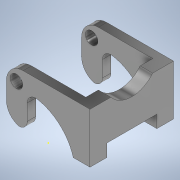
# Autodesk Inventor part: Peça 9
Saved by Autodesk Inventor 2021 (Build 250183000, 183)
## iProperties
Created: 2020-11-15
Part Number: Peça 9
Material: Liga de Nickel-Copper 400
Document SubType Name: Modeling
Designer: Bruno
Density: 8.83 g/cm^3
Appearance: Cromado - Preto polido
Author: Bruno
Autodesk Inventor part; units mm, degrees
ref_plane "YZ Plane" through (0, 0, 0) normal (1, 0, 0) x (0, 1, 0)
ref_plane "XZ Plane" through (0, 0, 0) normal (0, 1, 0) x (-1, 0, 0)
ref_plane "XY Plane" through (0, 0, 0) normal (0, 0, 1) x (1, 0, 0)
sketch "Esboço1" plane through (0, 0, 0) normal (0, 1, 0) x (-1, 0, 0)
  line L0 (-5, 5) -> (5, 5)
  line L1 (5, 5) -> (5, -5)
  line L2 (5, -5) -> (-5, -5)
  line L3 (-5, -5) -> (-5, 5)
  line L4 (-5, 5) -> (5, -5) construction
  line L5 (5, 5) -> (-5, -5) construction
  point P0 (0, 0)
  dimension "d0" = 10
  dimension "d1" = 10
  constraints: 12 end point, 2 midpoint, 2 parallel, 1 horizontal, 1 perpendicular
  measures "d0" distance between parallel lines of L2 L0
  measures "d1" distance between parallel lines of L3 L1
extrude "Extrusão1" add sketch "Esboço1" along normal blind 6
sketch "Esboço2" plane through (5, 0, 5) normal (1, 0, 0) x (0, 0, -1)
  line L0 (2, 0) -> (2, 1.5)
  line L1 (0, 0) -> (0, 6) projected
  line L2 (2, 1.5) -> (8, 1.5)
  line L3 (8, 1.5) -> (8, 0)
  line L4 (10, 0) -> (10, 6) projected
  line L5 (0, 0) -> (10, 0) projected
  point P0 (5, 0)
  dimension "d4" = 2
  dimension "d5" = 1.5
  dimension "d6" = 2
  dimension "d7" = 1.5
  constraints: 6 end point, 1 horizontal, 1 perpendicular, 1 vertical
  measures "d4" distance between parallel lines of L1 L0
  measures "d5" distance of L0.start L0.end
  measures "d6" distance between parallel lines of L4 L3
  measures "d7" distance between parallel lines of L5 L2
extrude "Extrusão2" cut sketch "Esboço2" against normal through all
sketch "Esboço3" plane through (-5, 0, 5) normal (0, 0, 1) x (1, 0, 0)
  line L0 (10, 0) -> (0, 0) projected
  arc A0 (8, 0) -> (2.5, 3.9823) centre (2.7087, -1.5186) ccw
  line L1 (0, 0) -> (0, 6) projected
  line L2 (2.5, 3.9823) -> (2.5, 0)
  point P0 (5, 0)
  dimension "d10" = 2
  dimension "d11" = 2.5
  dimension "d12" = 5.5049
  dimension "d13" = 2.7087
  constraints: 2 end point, 2 point on circle, 2 point on line, 1 centre point, 1 perpendicular
  measures "d10" distance of L0.start A0.start
  measures "d11" distance from line of L2.start L1
  measures "d12" radius of A0
  measures "d13" horizontal distance of L0.end A0.centre
extrude "Extrusão3" cut sketch "Esboço3" against normal through all
sketch "Esboço4" plane through (-5, 6, 5) normal (0, 0, 1) x (1, 0, 0)
  point P0 (5, -6)
fillet "Arredondamento1" radius 1 1 edges at (-2.5, 3.9823, 0)
fillet "Arredondamento2" radius 1 2 edges at (-2.5, 0, 4) (-2.5, 0, -4)
fillet "Arredondamento3" radius 2 3 edges at (-5, 6, 0) (-5, 0, -4) (-5, 0, 4)
sketch "Esboço5" plane through (5, 0, 5) normal (0, 0, 1) x (1, 0, 0)
  circle A0 centre (-8.8, 4.5) radius 0.75
  line L0 (0, 0) -> (0, 6) projected
  point P0 (-5, 0)
  dimension "d19" = 1.5
  dimension "d20" = 8.8
  dimension "d21" = 4.5
  constraints: 1 centre point
  measures "d19" diameter of A0
  measures "d20" distance from line of L0 A0.centre
  measures "d21" vertical distance of point (-5, 0) A0.centre
extrude "Extrusão4" cut sketch "Esboço5" against normal through all
sketch "Esboço6" plane through (0, 6, 0) normal (0, 1, 0) x (1, 0, 0)
  line L0 (-5, 5) -> (-5, -5) projected
  line L1 (-5, 4) -> (3.5, 4)
  line L2 (5, -5) -> (5, 5) projected
  line L3 (3.5, -4) -> (-5, -4)
  line L4 (-5, -4) -> (-5, 4)
  line L5 (5, 5) -> (-3, 5) projected
  line L6 (-3, -5) -> (5, -5) projected
  line L7 (3.5, 4) -> (3.5, -4)
  point P0 (0, 0)
  dimension "d24" = 1
  dimension "d25" = 1
  dimension "d26" = 1.5
  constraints: 8 end point, 2 perpendicular, 2 point on line, 1 horizontal
  measures "d24" distance between parallel lines of L1 L5
  measures "d25" distance between parallel lines of L6 L3
  measures "d26" distance between parallel lines of L2 L7
extrude "Extrusão5" cut sketch "Esboço6" against normal through all
sketch "Esboço7" plane through (5, 0, -5) normal (1, 0, 0) x (0, 0, -1)
  line L0 (-1, 6) -> (-9, 6) projected
  arc A0 (-7.5, 6) -> (-2.5, 6) centre (-5, 7.9975) ccw
  line L1 (-10, 0) -> (-10, 6) projected
  line L2 (0, 0) -> (0, 6) projected
  point P0 (-5, 0)
  dimension "d29" = 3.2
  dimension "d30" = 2.5
  dimension "d31" = 2.5
  constraints: 2 point on circle, 2 point on line, 1 centre point
  measures "d29" radius of A0
  measures "d30" distance from line of L1 A0.start
  measures "d31" distance from line of L2 A0.end
extrude "Extrusão6" cut sketch "Esboço7" against normal blind 6
